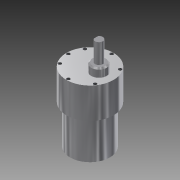
# Autodesk Inventor part: motor_polulu
Saved by Autodesk Inventor 2014 (Build 180170000, 170)
## iProperties
Created: 2014-11-03
Part Number: motor_polulu
Material: Generic
Document SubType Name: Sheet Metal
Designer: Gabriel
Density: 1 g/cm^3
Sheet Metal Rule: Default_mm
Appearance: Default
Author: Gabriel
Autodesk Inventor part; units mm, degrees
ref_plane "YZ Plane" through (0, 0, 0) normal (1, 0, 0) x (0, 1, 0)
ref_plane "XZ Plane" through (0, 0, 0) normal (0, 1, 0) x (-1, 0, 0)
ref_plane "XY Plane" through (0, 0, 0) normal (0, 0, 1) x (1, 0, 0)
sketch "Sketch1" plane through (0, 0, 0) normal (0, 0, 1) x (1, 0, 0)
  circle A0 centre (0, 0) radius 15.5
  dimension "d0" = 31
  constraints: 1 centre point, 1 coincident
  measures "d0" diameter of A0
extrude "Extrusion1" add sketch "Sketch1" along normal blind 30
sketch "Sketch2" plane through (0, 0, 30) normal (0, 0, 1) x (1, 0, 0)
  circle A0 centre (0, 0) radius 18.4
  dimension "d3" = 36.8
  constraints: 1 centre point, 1 coincident
  measures "d3" diameter of A0
extrude "Extrusion2" add sketch "Sketch2" along normal blind 24
sketch "Sketch3" plane through (0, 0, 54) normal (0, 0, 1) x (1, 0, 0)
  line L0 (0, 0) -> (7, 0)
  circle A0 centre (7, 0) radius 3
  circle A1 centre (7, 0) radius 6
  dimension "d6" = 7
  dimension "d7" = 6
  dimension "d8" = 12
  constraints: 2 centre point, 2 coincident, 2 end point, 1 horizontal
  measures "d6" distance of L0.start L0.end
  measures "d7" diameter of A0
  measures "d8" diameter of A1
extrude "Extrusion3" add sketch "Sketch3" along normal blind 22 contours A0
extrude "Extrusion4" add sketch "Sketch3" along normal blind 6.5
chamfer "Chamfer1" distance 1 angle 45 1 edges at (1, 0, 60.5)
sketch "Sketch4" plane through (7, 0, 76) normal (0, 0, 1) x (1, 0, 0)
  point P0 (-7, 0)
sketch "Sketch5" plane through (7, 0, 76) normal (0, 0, 1) x (1, 0, 0)
  line L0 (0, 0) -> (-2.4, 0)
  line L1 (-2.4, 0) -> (-2.4, -1.7999)
  line L2 (-2.4, 0) -> (-2.4, 1.8068)
  arc A0 (-2.4, 1.8068) -> (-2.4, -1.7999) centre (-0.0145, 0.0034) ccw
  point P0 (-7, 0)
  dimension "d16" = 2.4
  constraints: 6 end point, 2 point on circle, 1 centre point, 1 collinear, 1 horizontal, 1 perpendicular
  measures "d16" distance of L0.start L0.end
extrude "Extrusion5" cut sketch "Sketch5" against normal blind 12
sketch "Sketch6" plane through (4.6, -1.7999, 76) normal (-1, 0, 0) x (0, 0, 1)
  line L0 (-11.9968, 1.7999) -> (-7.9968, 1.7999)
  circle A0 centre (-7.9968, 1.7999) radius 0.5
  point P0 (-76, 1.7999)
  dimension "d19" = 4
  dimension "d20" = 1
  constraints: 2 end point, 1 centre point, 1 coincident, 1 horizontal
  measures "d19" distance of L0.start L0.end
  measures "d20" diameter of A0
sketch "Sketch8" plane through (0, 0, 54) normal (0, 0, 1) x (1, 0, 0)
  point P0 (0, 0)
sketch "Sketch9" plane through (0, 0, 54) normal (0, 0, 1) x (1, 0, 0)
  line L0 (0, 0) -> (0, 16.95)
  circle A0 centre (0, 16.95) radius 1.25
  line L1 (0, 0) -> (0, -16.95)
  circle A1 centre (0, -16.95) radius 1.25
  line L2 (0, 0) -> (-16.95, 0)
  circle A2 centre (-16.95, 0) radius 1.25
  line L3 (0, -16.95) -> (-13.7744, -9.8425)
  circle A3 centre (-13.7744, -9.8425) radius 1.25
  circle A4 centre (-13.7744, 9.8425) radius 1.25
  line L4 (0, 16.95) -> (-13.7744, 9.8425)
  line L5 (-13.7744, -9.8425) -> (-13.7744, 9.8425)
  line L6 (0, -16.95) -> (13.7744, -9.8425)
  circle A5 centre (13.7744, -9.8425) radius 1.25
  line L7 (0, 16.95) -> (13.7744, 9.8425)
  circle A6 centre (13.7744, 9.8425) radius 1.25
  line L8 (0, 0) -> (13.7744, 0)
  line L9 (13.7744, 0) -> (13.7744, -9.8425)
  dimension "d49" = 16.95
  dimension "d50" = 2.5
  dimension "d51" = 16.95
  dimension "d52" = 2.5
  dimension "d66" = 16.95
  dimension "d67" = 2.5
  dimension "d68" = 15.5
  dimension "d69" = 2.5
  dimension "d71" = 2.5
  dimension "d72" = 15.5
  dimension "d116" = 2.5
  dimension "d117" = 2.5
  constraints: 20 end point, 7 centre point, 6 coincident, 4 perpendicular, 3 equal length, 1 vertical
  measures "d49" distance of L0.start L0.end
  measures "d50" diameter of A0
  measures "d51" distance of L0.start L1.end
  measures "d52" diameter of A1
  measures "d66" distance of L0.start L2.end
  measures "d67" diameter of A2
  measures "d68" distance of L3.start L3.end
  measures "d69" diameter of A3
  measures "d71" diameter of A4
  measures "d72" distance of L4.start L4.end
  measures "d116" diameter of A5
  measures "d117" diameter of A6
hole "Hole2" at (0, -16.95, 54) direction (0, 0, -1) diameter 2.5 end through all
extrude "Extrusion9" cut sketch "Sketch9" against normal through all contours A0 L4 L0 | L0 L7 A0 | L4 A0 L7
thread "Thread5" size "M3x0.5" class "6H" standard "ANSI Metric M Profile" full length
thread "Thread6" size "M3x0.5" class "6H" standard "ANSI Metric M Profile" full length
hole "Hole3" at (-13.7744, -9.8425, 54) direction (0, 0, -1) diameter 2.5 end through all
hole "Hole4" at (-13.7744, 9.8425, 54) direction (0, 0, -1) diameter 2.5 end through all
thread "Thread7" size "M3x0.5" class "6H" standard "ANSI Metric M Profile" full length
thread "Thread8" size "M3x0.5" class "6H" standard "ANSI Metric M Profile" full length
hole "Hole7" at (-16.95, 0, 54) direction (0, 0, -1) diameter 2.5 end through all
thread "Thread9" size "M3x0.5" class "6H" standard "ANSI Metric M Profile" length 10
hole "Hole8" at (13.7744, -9.8425, 54) direction (0, 0, -1) diameter 2.5 end through all
hole "Hole9" at (13.7744, 9.8425, 54) direction (0, 0, -1) diameter 2.5 end through all
thread "Thread10" size "M3x0.5" class "6H" standard "ANSI Metric M Profile" full length
thread "Thread11" size "M2.5x0.45" class "6H" standard "ANSI Metric M Profile" full length
thread "Thread12" size "M3x0.5" class "6H" standard "ANSI Metric M Profile" full length
equation "\"d58\" = Thickness"
equation "\"d78\" = Thickness"
equation "\"d85\" = Thickness"
equation "\"d110\" = Thickness"
equation "\"d123\" = Thickness"
equation "\"d130\" = Thickness"
equation "\"BendRadius\" = Thickness"
equation "\"BendReliefWidth\" = Thickness"
equation "\"BendReliefDepth\" = 0.5 * Thickness"
equation "\"CornerReliefSize\" = 4 * Thickness"
equation "\"MinimumRemnant\" = 2 * Thickness"
equation "\"TransitionRadius\" = BendRadius"
equation "\"JacobiRadiusSize\" = BendRadius"
equation "\"GapSize\" = Thickness"
equation "\"Thickness\" = 0.5"
body "Solid1"
